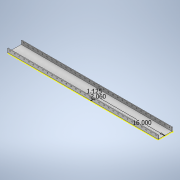
# Autodesk Inventor part: AM14U4_Plate
Saved by Autodesk Inventor 2020.3 (Build 243373000, 373)
## iProperties
Created: 2020-09-23
Part Number: AM14U4_Plate
Material: Generic
Document SubType Name: Modeling
Designer: super
Density: 1 g/cm^3
Appearance: Default
Author: super
Autodesk Inventor part; units mm, degrees
ref_plane "YZ Plane" through (0, 0, 0) normal (1, 0, 0) x (0, 1, 0)
ref_plane "XZ Plane" through (0, 0, 0) normal (0, 1, 0) x (-1, 0, 0)
ref_plane "XY Plane" through (0, 0, 0) normal (0, 0, 1) x (1, 0, 0)
sketch "Sketch1" plane through (0, 0, 0) normal (1, 0, 0) x (0, 1, 0)
  line L0 (0, 0) -> (-22.225, 0)
  line L1 (-22.225, 0) -> (-22.225, 77.724)
  line L2 (-22.225, 77.724) -> (0, 77.724)
  line L3 (0, 77.724) -> (0, 74.422)
  line L4 (0, 74.422) -> (-18.923, 74.422)
  line L5 (-18.923, 74.422) -> (-18.923, 3.302)
  line L6 (-18.923, 3.302) -> (0, 3.302)
  line L7 (0, 3.302) -> (0, 0)
  dimension "d0" = 22.225
  dimension "d1" = 77.724
  dimension "d2" = 3.302
  dimension "d3" = 18.923
  dimension "d4" = 71.12
  constraints: 16 end point, 7 perpendicular, 1 horizontal, 1 point on line
  measures "d0" distance of L0.start L0.end
  measures "d1" distance of L0.end L1.end
  measures "d2" distance of L2.end L3.end
  measures "d3" distance of L3.end L4.end
  measures "d4" distance of L4.end L5.end
extrude "Extrusion1" add sketch "Sketch1" against normal blind 812.8
fillet "Fillet1" radius 3.175 1 edges at (-406.4, -22.225, 0)
fillet "Fillet2" radius 3.175 1 edges at (-406.4, -22.225, 77.724)
sketch "Sketch2" plane through (0, 0, 0) normal (0, 0, -1) x (-1, 0, 0)
  circle A0 centre (12.7, -6.35) radius 2.667
  point P0 (0, 0)
  dimension "d11" = 5.334
  constraints: 1 centre point
  measures "d11" diameter of A0
extrude "Extrusion2" cut sketch "Sketch2" against normal blind 3.302
pattern_linear "Rectangular Pattern1" count 32 spacing 25.4 along (-1, 0, 0) of "Extrusion2"
sketch "Sketch3" plane through (-812.8, 0, 77.724) normal (0, 0, 1) x (1, 0, 0)
  line L0 (812.8, -18.923) -> (812.8, 0) projected
  circle A0 centre (800.1, -6.35) radius 2.667
  dimension "d19" = 5.334
  constraints: 1 centre point
  measures "d19" diameter of A0
extrude "Extrusion3" cut sketch "Sketch3" against normal blind 3.302
pattern_linear "Rectangular Pattern2" count 32 spacing 25.4 along (-1, 0, 0) of "Extrusion3"
sketch "Sketch4" plane through (-812.8, -22.225, 3.175) normal (0, -1, 0) x (1, 0, 0)
  circle A0 centre (406.4, 22.225) radius 14.2862
  line L0 (812.8, 71.374) -> (812.8, 0) projected
  line L1 (812.8, 74.549) -> (0, 74.549) projected
  point P0 (812.8, -3.175)
  dimension "d25" = 28.5725
  dimension "d26" = 406.4
  dimension "d27" = 52.324
  constraints: 1 centre point
  measures "d25" diameter of A0
  measures "d26" distance from line of L0 A0.centre
  measures "d27" distance from line of L1 A0.centre
body "Solid1"
